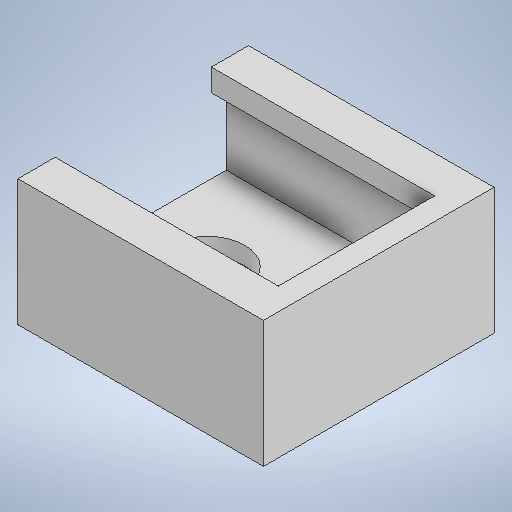
# Autodesk Inventor part: LuftSensorHållare
Saved by Autodesk Inventor 2025.2 (Build 292293000, 293)
## iProperties
Created: 2025-01-23
Part Number: LuftSensorHållare
Material: Generic
Document SubType Name: Modeling
Designer: 24oscnor
Density: 1 g/cm^3
Appearance: Default
Author: 24oscnor
Autodesk Inventor part; units mm, degrees
ref_plane "YZ Plane" through (0, 0, 0) normal (1, 0, 0) x (0, 1, 0)
ref_plane "XZ Plane" through (0, 0, 0) normal (0, 1, 0) x (-1, 0, 0)
ref_plane "XY Plane" through (0, 0, 0) normal (0, 0, 1) x (1, 0, 0)
sketch "Sketch1" plane through (0, 0, 0) normal (0, 1, 0) x (-1, 0, 0)
  line L0 (0, 0) -> (15, 0)
  line L1 (15, 0) -> (15, 12.5)
  line L2 (15, 12.5) -> (0, 12.5)
  line L3 (0, 12.5) -> (0, 0)
  dimension "d0" = 15
  dimension "d1" = 12.5
  constraints: 8 end point, 2 parallel, 1 horizontal, 1 perpendicular
  measures "d0" distance of L0.start L0.end
  measures "d1" distance of L2.end L0.start
extrude "Extrusion1" add sketch "Sketch1" along normal blind 2
sketch "Sketch2" plane through (-15, 0, 12.5) normal (0, 0, 1) x (1, 0, 0)
  line L0 (0, 0) -> (15, 0)
  line L1 (15, 0) -> (15, 8.5)
  line L2 (15, 8.5) -> (0, 8.5)
  line L3 (0, 8.5) -> (0, 0)
  point P0 (15, 0)
  dimension "d4" = 8.5
  dimension "d5" = 15
  constraints: 8 end point, 2 parallel, 1 horizontal, 1 perpendicular
  measures "d4" distance of L0.end L1.end
  measures "d5" distance of L0.start L0.end
extrude "Extrusion2" add sketch "Sketch2" along normal blind 1.5
sketch "Sketch3" plane through (0, 0, 0) normal (1, 0, 0) x (0, 0, -1)
  line L0 (-14, 8.5) -> (-14, 0) projected
  line L1 (-14, 8.5) -> (0, 8.5)
  line L2 (0, 8.5) -> (0, 0)
  line L3 (0, 0) -> (-14, 0)
  line L4 (-14, 0) -> (-14, 8.5)
  point P0 (-14, 0)
  constraints: 8 end point, 2 parallel, 1 horizontal, 1 perpendicular
extrude "Extrusion3" add sketch "Sketch3" along normal blind 1.5
sketch "Sketch4" plane through (-15, 0, 12.5) normal (0, 0, -1) x (-1, 0, 0)
  line L0 (-15, 8.5) -> (0, 8.5) projected
  line L1 (-15, 2) -> (-15, 8.5) projected
  line L2 (0, 8.5) -> (-15, 8.5)
  line L3 (-15, 8.5) -> (-15, 7)
  line L4 (-15, 7) -> (0, 7)
  line L5 (0, 7) -> (0, 8.5)
  point P0 (-15, 0)
  dimension "d11" = 1.5
  constraints: 8 end point, 2 parallel, 1 horizontal, 1 perpendicular, 1 point on line
  measures "d11" distance between parallel lines of L4 L0
extrude "Extrusion4" add sketch "Sketch4" along normal blind 1
sketch "Sketch5" plane through (0, 2, 0) normal (0, 1, 0) x (1, 0, 0)
  circle A0 centre (-10, -6.25) radius 2.5
  line L0 (-15, 0) -> (-15, -12.5) projected
  line L1 (-15, -14) -> (1.5, -14) projected
  point P0 (0, 0)
  dimension "d14" = 5
  dimension "d15" = 5
  dimension "d28" = 7.75
  constraints: 1 centre point
  measures "d14" diameter of A0
  measures "d15" distance from line of L0 A0.centre
  measures "d28" distance from line of A0.centre L1
extrude "Extrusion5" cut sketch "Sketch5" against normal blind 1.2
sketch "Sketch6" plane through (-10, 0.8, 6.25) normal (0, 1, 0) x (1, 0, 0)
  circle A0 centre (0, 0) radius 2.5 projected
  circle A1 centre (0, 0) radius 1.5
  point P0 (10, 6.25)
  dimension "d29" = 3
  constraints: 1 centre point, 1 coincident
  measures "d29" diameter of A1
extrude "Extrusion6" cut sketch "Sketch6" against normal blind 1.2 contours A1
sketch "Sketch7" plane through (-15, 0, 0) normal (0, 0, -1) x (-1, 0, 0)
  line L0 (-16.5, 0) -> (0, 0)
  line L1 (0, 0) -> (0, 2)
  line L2 (0, 2) -> (-16.5, 2)
  line L3 (-16.5, 2) -> (-16.5, 0)
  line L4 (-15, 8.5) -> (-16.5, 8.5) projected
  line L5 (-16.5, 2) -> (-15, 2)
  line L6 (-15, 2) -> (-15, 8.5)
  line L7 (-15, 8.5) -> (-16.5, 8.5)
  line L8 (-16.5, 8.5) -> (-16.5, 2)
  line L9 (0, 8.5) -> (-15, 8.5) projected
  line L10 (-15, 2) -> (0, 2)
  line L11 (0, 2) -> (0, 8.5)
  line L12 (0, 8.5) -> (-15, 8.5)
  line L13 (-15, 8.5) -> (-15, 2)
  point P0 (-15, 0)
  constraints: 24 end point, 6 parallel, 3 horizontal, 3 perpendicular
extrude "Extrusion7" add sketch "Sketch7" along normal blind 1.5
sketch "Sketch8" plane through (-15, 0, 0) normal (0, 0, 1) x (1, 0, 0)
  line L0 (0, 8.5) -> (15, 8.5) projected
  line L1 (0, 8.5) -> (15, 8.5)
  line L2 (15, 8.5) -> (15, 7)
  line L3 (15, 7) -> (0, 7)
  line L4 (0, 7) -> (0, 8.5)
  point P0 (15, 0)
  dimension "d25" = 1.5
  constraints: 8 end point, 2 parallel, 1 horizontal, 1 perpendicular
  measures "d25" distance between parallel lines of L0 L3
extrude "Extrusion8" add sketch "Sketch8" along normal blind 1
body "Solid1"
